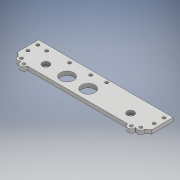
# Autodesk Inventor part: 5枚目
Saved by Autodesk Inventor 2018 (Build 220112000, 112)
## iProperties
Created: 2018-08-16
Part Number: 5枚目
Material: 一般
Document SubType Name: Modeling
Designer: shun2
Density: 1 g/cm^3
Appearance: 既定
Author: shun2
Autodesk Inventor part; units mm, degrees
ref_plane "YZ Plane" through (0, 0, 0) normal (1, 0, 0) x (0, 1, 0)
ref_plane "XZ Plane" through (0, 0, 0) normal (0, 1, 0) x (-1, 0, 0)
ref_plane "XY Plane" through (0, 0, 0) normal (0, 0, 1) x (1, 0, 0)
sketch "スケッチ1" plane through (0, 0, 0) normal (0, 0, 1) x (1, 0, 0)
  circle A0 centre (179.6946, 9.9994) radius 2.15
  circle A1 centre (10.6603, 9.9994) radius 2.15
  circle A2 centre (100.6774, 40.6494) radius 2.15
  circle A3 centre (80.1774, 38.4994) radius 2.15
  circle A4 centre (50.1774, 38.4994) radius 2.15
  circle A5 centre (171.2766, 4.9994) radius 2.15
  circle A6 centre (19.0782, 4.9994) radius 2.15
  circle A7 centre (19.2933, 37.0055) radius 2.15
  circle A8 centre (184.5394, 23.9994) radius 2.15
  circle A9 centre (184.5394, 37.9994) radius 2.15
  circle A10 centre (5.8155, 23.9994) radius 2.15
  circle A11 centre (5.8155, 37.9994) radius 2.15
  line L0 (190.3548, 44.9994) -> (190.3548, 14.9994)
  line L1 (190.3548, 14.9994) -> (184.6641, 10.5508)
  arc A12 (176.6082, 6.0657) -> (184.6641, 10.5508) centre (179.6946, 9.9994) ccw
  line L2 (176.6085, 6.0658) -> (176.2124, 5.8452)
  arc A13 (166.3265, 4.9994) -> (176.2508, 5.8665) centre (171.3265, 4.9994) ccw
  line L3 (166.2766, 4.9994) -> (24.0782, 4.9994)
  arc A14 (14.154, 5.8665) -> (24.0782, 4.9994) centre (19.0782, 4.9994) ccw
  line L4 (14.154, 5.8665) -> (13.7466, 6.0657)
  arc A15 (5.6908, 10.5508) -> (13.7466, 6.0657) centre (10.6603, 9.9994) ccw
  line L5 (5.6908, 10.5508) -> (0, 14.9994)
  line L6 (0, 14.9994) -> (0, 44.9994)
  line L7 (0, 44.9994) -> (190.3548, 44.9994)
  circle A16 centre (155.1774, 19.9994) radius 5
  circle A17 centre (155.1774, 19.9994) radius 18
  circle A18 centre (95.1774, 19.9994) radius 18
  circle A19 centre (65.1774, 19.9994) radius 18
  circle A20 centre (35.1774, 19.9994) radius 18
  circle A21 centre (35.1774, 19.9994) radius 5
  circle A22 centre (65.1774, 19.9994) radius 9.5
  circle A23 centre (95.1774, 19.9994) radius 9.5
  line L8 (0, 44.9994) -> (190.3548, 44.9994)
  line L9 (190.3548, 14.9994) -> (190.3548, 44.9994)
  line L10 (184.6641, 10.5508) -> (190.3548, 14.9994)
  line L11 (0, 14.9994) -> (0, 44.9994)
  line L12 (5.6908, 10.5508) -> (0, 14.9994)
  line L13 (13.7466, 6.0657) -> (14.154, 5.8665)
  line L14 (24.0782, 4.9994) -> (166.3265, 4.9994)
  line L15 (176.6085, 6.0658) -> (176.2508, 5.8665)
  arc A24 (5.6908, 10.5508) -> (13.7466, 6.0657) centre (10.6603, 9.9994) ccw
  arc A25 (14.154, 5.8665) -> (24.0782, 4.9994) centre (19.0782, 4.9994) ccw
  arc A26 (176.6085, 6.0658) -> (184.6641, 10.5508) centre (179.6948, 9.9993) ccw
  arc A27 (166.3265, 4.9994) -> (176.2508, 5.8665) centre (171.3265, 4.9994) ccw
  circle A28 centre (5.8155, 37.9994) radius 2.15
  circle A29 centre (5.8155, 23.9994) radius 2.15
  circle A30 centre (10.6603, 9.9994) radius 2.15
  circle A31 centre (19.0782, 4.9994) radius 2.15
  circle A32 centre (19.2933, 37.0055) radius 2.15
  circle A33 centre (50.1774, 38.4994) radius 2.15
  circle A34 centre (80.1774, 38.4994) radius 2.15
  circle A35 centre (100.6774, 40.6494) radius 2.15
  circle A36 centre (184.5394, 37.9994) radius 2.15
  circle A37 centre (184.5394, 23.9994) radius 2.15
  circle A38 centre (179.6948, 9.9993) radius 2.1498
  circle A39 centre (171.3265, 4.9994) radius 2.1001
  circle A40 centre (35.1774, 19.9994) radius 5
  circle A41 centre (65.1774, 19.9994) radius 9.5
  circle A42 centre (95.1774, 19.9994) radius 9.5
  circle A43 centre (155.1774, 19.9994) radius 5
  point P0 (0, 0)
  constraints: 44 centre point, 32 end point, 19 point on circle, 16 coincident, 16 concentric, 6 collinear, 1 horizontal, 1 point on line
extrude "押し出し1" add sketch "スケッチ1" along normal blind 5.5 contours L0 L1 A12 L2 A13 L14 L3 A17 A18 A19 A20 A14 L4 A15 L5 L6 L7 | L3 A17 | A20 A19 L3 | A20 A19 L3 | A20 A19 | A19 A18 L3 A20 | L3 A18 A19 | A19 A18 | L3 A19 A18 picked at (155.3783, 8.3449)
